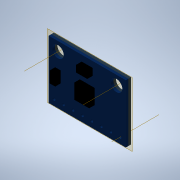
# Autodesk Inventor part: GY_521
Saved by Autodesk Inventor 2021 (Build 250183000, 183)
## iProperties
Created: 2020-08-26
Part Number: GY_521
Material: Generisch
Document SubType Name: Modeling
Designer: ALEX
Density: 1 g/cm^3
Appearance: Vorgabe
Mass: 0.469952 g
Surface Area: 8.23619 cm^2
Volume: 0.469952 cm^3
Author: ALEX
Autodesk Inventor part; units mm, degrees
ref_plane "YZ Plane" through (0, 0, 0) normal (1, 0, 0) x (0, 1, 0)
ref_plane "XZ Plane" through (0, 0, 0) normal (0, 1, 0) x (-1, 0, 0)
ref_plane "XY Plane" through (0, 0, 0) normal (0, 0, 1) x (1, 0, 0)
sketch "Skizze1" plane through (0, 0, 0) normal (0, 0, 1) x (1, 0, 0)
  line L0 (0, 0) -> (20.8, 0)
  line L1 (20.8, 0) -> (20.8, 15.7)
  line L2 (20.8, 15.7) -> (0, 15.7)
  line L3 (0, 15.7) -> (0, 0)
  circle A0 centre (2.5, 13.2) radius 1.55
  circle A1 centre (18.3, 13.2) radius 1.55
  dimension "d0" = 20.8
  dimension "d1" = 15.7
  dimension "d2" = 2.5
  dimension "d3" = 2.5
  dimension "d4" = 2.5
  dimension "d5" = 2.5
  dimension "d6" = 3.1
  dimension "d7" = 3.1
  constraints: 8 end point, 2 centre point, 2 parallel, 1 horizontal, 1 perpendicular
  measures "d0" distance of L1.end L2.end
  measures "d1" distance of L2.end L0.start
  measures "d2" distance from line of L2 A0.centre
  measures "d3" distance from line of L3 A0.centre
  measures "d4" distance from line of L2 A1.centre
  measures "d5" distance from line of L1 A1.centre
  measures "d6" diameter of A0
  measures "d7" diameter of A1
extrude "Grundkörper" add sketch "Skizze1" along normal blind 1.4
sketch "Skizze2" plane through (0, 0, 1.4) normal (0, 0, 1) x (1, 0, 0)
  line L0 (8.4, 5.7) -> (12.4, 5.7)
  line L1 (12.4, 5.7) -> (12.4, 9.7)
  line L2 (12.4, 9.7) -> (8.4, 9.7)
  line L3 (8.4, 9.7) -> (8.4, 5.7)
  line L4 (20.8, 0) -> (20.8, 15.7) projected
  line L5 (20.8, 15.7) -> (0, 15.7) projected
  line L6 (1.75, 6.2) -> (3.25, 6.2)
  line L7 (3.25, 6.2) -> (3.25, 9.2)
  line L8 (3.25, 9.2) -> (1.75, 9.2)
  line L9 (1.75, 9.2) -> (1.75, 6.2)
  line L10 (12.4, 7.7) -> (8.4, 7.7) construction
  line L11 (3.25, 7.7) -> (1.75, 7.7) construction
  line L12 (0, 15.7) -> (0, 0) construction
  line L13 (8.9, 14.1) -> (11.9, 14.1)
  line L14 (11.9, 14.1) -> (11.9, 12.3)
  line L15 (11.9, 12.3) -> (8.9, 12.3)
  line L16 (8.9, 12.3) -> (8.9, 14.1)
  line L17 (10.4, 15.7) -> (10.4, 0) construction
  line L18 (0, 0) -> (20.8, 0) construction
  line L19 (10.4, 9.7) -> (10.4, 5.7) construction
  circle A0 centre (2.5, 13.2) radius 1.55 construction
  circle A1 centre (18.3, 13.2) radius 1.55 construction
  line L20 (2.5, 13.2) -> (18.3, 13.2) construction
  line L21 (10.4, 14.1) -> (10.4, 12.3) construction
  line L22 (8.9, 13.2) -> (11.9, 13.2) construction
  line L23 (2.5, 13.2) -> (2.5, 11.65) construction
  line L24 (2.5, 9.2) -> (2.5, 6.2) construction
  dimension "d10" = 4
  dimension "d11" = 4
  dimension "d13" = 6
  dimension "d14" = 3
  dimension "d15" = 1.5
  dimension "d17" = 1.8
  dimension "d18" = 3
  constraints: 42 end point, 14 midpoint, 6 parallel, 5 collinear, 4 horizontal, 3 perpendicular, 1 vertical, 1 vertical alignment, 1 other
  measures "d10" distance of L2.end L0.start
  measures "d11" distance of L0.start L0.end
  measures "d13" distance between parallel lines of L5 L2
  measures "d14" distance of L6.end L7.end
  measures "d15" distance of L7.end L8.end
  measures "d17" distance of L15.end L13.start
  measures "d18" distance of L13.start L13.end
extrude "SMDs" add sketch "Skizze2" along normal blind 1.5
sketch "Skizze3" plane through (0, 0, 1.4) normal (0, 0, 1) x (1, 0, 0)
  line L0 (20.8, 15.7) -> (0, 15.7) construction
  line L1 (10.4, 15.7) -> (10.4, 0) construction
  line L2 (0, 0) -> (20.8, 0) construction
  line L3 (0, 15.7) -> (0, 0) construction
  line L4 (0, 1.6) -> (20.8, 1.6) construction
  line L5 (20.8, 0) -> (20.8, 15.7) construction
  point P0 (19.225, 1.6132)
  point P1 (16.685, 1.6132)
  point P2 (14.145, 1.6132)
  point P3 (11.605, 1.6132)
  point P4 (9.065, 1.6132)
  point P5 (6.525, 1.6132)
  point P6 (3.985, 1.6132)
  point P7 (1.445, 1.6132)
  dimension "d28" = 14.1
  dimension "d29" = 17.65
  dimension "d33" = 2.54
  constraints: 4 end point, 2 horizontal, 2 midpoint, 2 point on line, 7 other
  measures "d28" distance between parallel lines of L0 L4
  measures "d29" diameter of point (19.225, 1.613) L1
  measures "d33" distance of point (19.225, 1.613) point (16.685, 1.613)
hole "Bohrung1" at (19.225, 1.6132, 1.4) at (16.685, 1.6132, 1.4) at (14.145, 1.6132, 1.4) at (11.605, 1.6132, 1.4) at (9.065, 1.6132, 1.4) at (6.525, 1.6132, 1.4) at (3.985, 1.6132, 1.4) at (1.445, 1.6132, 1.4) direction (0, 0, -1) diameter 0.75 end through all
ref_plane "Work Plane1" through (0, 0, 0.7) normal (0, 0, 1) x (1, 0, 0)
